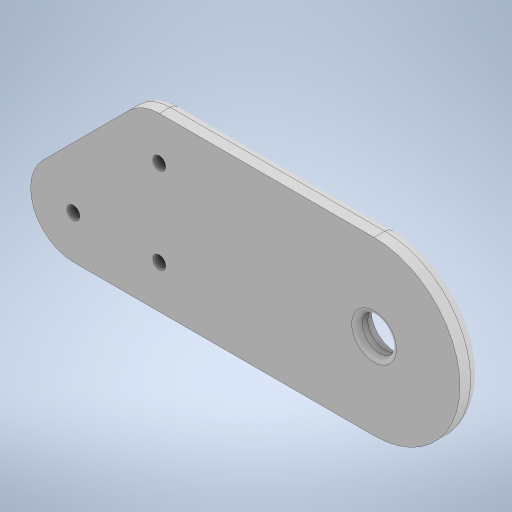
# Autodesk Inventor part: Bearing Bracket
Saved by Autodesk Inventor 2024 (Build 280153000, 153)
## iProperties
Created: 2024-01-19
Part Number: Bearing Bracket
Material: Generic
Document SubType Name: Modeling
Designer: CJ110
Density: 1 g/cm^3
Appearance: Default
Author: CJ110
Autodesk Inventor part; units mm, degrees
ref_plane "YZ Plane" through (0, 0, 0) normal (1, 0, 0) x (0, 1, 0)
ref_plane "XZ Plane" through (0, 0, 0) normal (0, 1, 0) x (-1, 0, 0)
ref_plane "XY Plane" through (0, 0, 0) normal (0, 0, 1) x (1, 0, 0)
sketch "Sketch1" plane through (0, 0, 0) normal (0, 0, 1) x (1, 0, 0)
  line L0 (0, 0) -> (127, 0)
  line L1 (127, 0) -> (127, 50.8)
  line L2 (127, 50.8) -> (0, 50.8)
  line L3 (0, 50.8) -> (0, 0)
  dimension "d0" = 127
  dimension "d1" = 50.8
  constraints: 8 end point, 2 parallel, 1 horizontal, 1 perpendicular
  measures "d0" distance between parallel lines of L3 L1
  measures "d1" distance between parallel lines of L0 L2
extrude "Extrusion1" add sketch "Sketch1" against normal blind 6.35
sketch "Sketch2" plane through (0, 0, -6.35) normal (0, 0, 1) x (1, 0, 0)
  line L0 (127, 0) -> (127, 50.8) projected
  line L1 (127, 50.8) -> (0, 50.8) projected
  line L2 (0, 50.8) -> (0, 0) projected
  line L3 (0, 0) -> (127, 0) projected
  line L4 (0, 25.4) -> (127, 25.4) construction
  circle A0 centre (12.7, 12.7) radius 1.905
  circle A1 centre (12.7, 12.7) radius 4.445
  circle A2 centre (38.1, 12.7) radius 1.905
  circle A3 centre (38.1, 12.7) radius 4.445
  circle A4 centre (38.1, 38.1) radius 1.905
  circle A5 centre (38.1, 38.1) radius 4.445
  line L5 (0, 17.9605) -> (32.8395, 50.8)
  line L6 (0, 0) -> (50.8, 50.8) construction
  circle A6 centre (38.1, 38.1) radius 12.7 construction
  dimension "d4" = 3.81
  dimension "d5" = 8.89
  dimension "d6" = 25.4
  dimension "d7" = 25.4
  dimension "d8" = 12.7
  dimension "d10" = 12.7
  constraints: 7 centre point, 6 end point, 4 coincident, 4 equal radius, 4 point on line, 2 midpoint, 2 tangent, 1 horizontal, 1 horizontal alignment, 1 parallel, 1 vertical alignment
  measures "d4" diameter of A4
  measures "d5" diameter of A5
  measures "d6" distance of A0.centre A2.centre
  measures "d7" distance of A2.centre A4.centre
  measures "d8" distance from line of L4 A0.centre
  measures "d10" distance from line of L2 A0.centre
extrude "Extrusion2" cut sketch "Sketch2" along normal through all contours L5 L2 L1 | A0 | A2 | A4
extrude "Extrusion3" cut sketch "Sketch2" along normal blind 3.175 contours A1 | A3 | A5
sketch "Sketch7" plane through (0, 0, -6.35) normal (0, 0, -1) x (-1, 0, 0)
  circle A0 centre (-101.6, 25.4) radius 7.239
  circle A1 centre (-101.6, 25.4) radius 5.08
  circle A2 centre (-101.6, 38.1) radius 1.143
  circle A3 centre (-101.6, 12.7) radius 1.143
  circle A4 centre (-38.1, 12.7) radius 4.445 projected
  circle A5 centre (-12.7, 12.7) radius 4.445 projected
  circle A6 centre (-38.1, 38.1) radius 4.445 projected
  line L0 (0, 17.9605) -> (-32.8395, 50.8) projected
  line L1 (-32.8395, 50.8) -> (-127, 50.8) projected
  line L2 (-127, 50.8) -> (-127, 0) projected
  line L3 (-127, 0) -> (0, 0) projected
  line L4 (0, 0) -> (0, 17.9605) projected
  line L5 (-127, 25.4) -> (-7.4395, 25.4) construction
  line L6 (-101.6, 50.8) -> (-101.6, 0) construction
  dimension "d40" = 25.4
  dimension "d41" = 14.478
  dimension "d42" = 10.16
  dimension "d43" = 2.286
  dimension "d44" = 12.7
  dimension "d45" = 12.7
  constraints: 6 point on line, 4 centre point, 4 end point, 2 midpoint, 1 coincident, 1 equal radius, 1 horizontal, 1 perpendicular
  measures "d40" distance from line of A0.centre L2
  measures "d41" diameter of A0
  measures "d42" diameter of A1
  measures "d43" diameter of A2
  measures "d44" distance from line of L5 A2.centre
  measures "d45" distance from line of L5 A3.centre
extrude "Extrusion9" cut sketch "Sketch7" against normal through all contours A1
extrude "Extrusion10" cut sketch "Sketch7" against normal blind 3.175 contours A0 | A2 | A3
sketch "Sketch8" plane through (0, 0, -6.35) normal (0, 0, -1) x (-1, 0, 0)
  circle A0 centre (-101.6, 25.4) radius 7.239 projected
  circle A1 centre (-101.6, 12.7) radius 1.143 projected
  circle A2 centre (-101.6, 38.1) radius 1.143 projected
  circle A3 centre (-38.1, 12.7) radius 4.445 projected
  circle A4 centre (-12.7, 12.7) radius 4.445 projected
  circle A5 centre (-38.1, 38.1) radius 4.445 projected
  line L0 (0, 17.9605) -> (-32.8395, 50.8) projected
  line L1 (-32.8395, 50.8) -> (-127, 50.8) projected
  line L2 (-127, 50.8) -> (-127, 0) projected
  line L3 (-127, 0) -> (0, 0) projected
  line L4 (0, 0) -> (0, 17.9605) projected
  circle A6 centre (-38.1, 38.1) radius 12.7
  circle A7 centre (-12.7, 12.7) radius 12.7
  circle A8 centre (-101.6, 25.4) radius 25.4
  point P0 (-3.7197, 21.6803)
  point P1 (0, 12.7)
  point P2 (-12.7, 0)
  point P3 (-38.1, 50.8)
  point P4 (-29.1197, 47.0803)
  point P5 (-127, 25.4)
  point P6 (-101.6, 50.8)
  point P7 (-101.6, 0)
  constraints: 3 centre point, 3 coincident, 3 tangent
extrude "Extrusion11" cut sketch "Sketch8" against normal through all contours L4 A7 L0 | L4 L3 A7 | A6 L1 L0 | L3 L2 A8 | A8 L2 L1
fillet "Fillet5" radius 1.5875 3 edges at (33.655, 38.1, -6.35) (33.655, 12.7, -6.35) (8.255, 12.7, -6.35)
fillet "Fillet6" radius 1.5875 1 edges at (106.68, 25.4, 0)
fillet "Fillet7" radius 3.175 6 edges at (127, 25.4, -6.35) (57.15, 0, -6.35) (0.9667, 7.8399, -6.35) (16.4197, 34.3803, -6.35) (33.2399, 49.8333, -6.35) (69.85, 50.8, -6.35)
equation "\"d45\" = d44"
body "Solid1"
